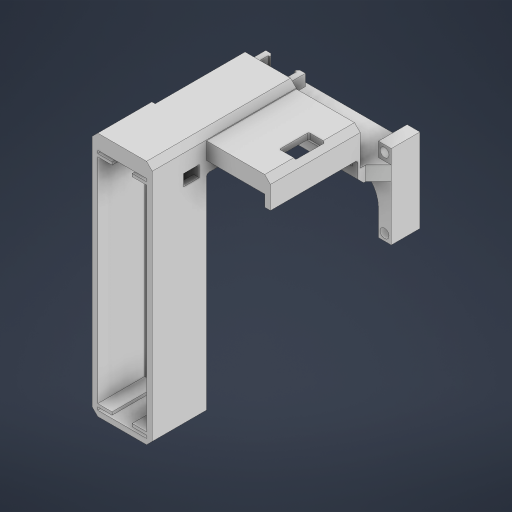
# Autodesk Inventor part: ElectronicsMount
Saved by Autodesk Inventor 2024.1 (Build 281209000, 209)
## iProperties
Created: 2023-11-16
Part Number: ElectronicsMount
Material: Generic
Document SubType Name: Modeling
Designer: Brandon
Density: 1 g/cm^3
Appearance: Default
Author: Brandon
Autodesk Inventor part; units mm, degrees
ref_plane "YZ Plane" through (0, 0, 0) normal (1, 0, 0) x (0, 1, 0)
ref_plane "XZ Plane" through (0, 0, 0) normal (0, 1, 0) x (-1, 0, 0)
sketch "Sketch1" plane through (0, 0, 0) normal (0, 0, 1) x (1, 0, 0)
  line L0 (-22, -8.75) -> (-22, 8.75) projected
  arc A0 (-22, -8.75) -> (-21.5, -9.25) centre (-21.5, -8.75) ccw projected
  line L1 (21.5, -9.25) -> (-21.5, -9.25) projected
  arc A1 (21.5, -9.25) -> (22, -8.75) centre (21.5, -8.75) ccw projected
  line L2 (22, 8.75) -> (22, -8.75) projected
  arc A2 (22, 8.75) -> (21.5, 9.25) centre (21.5, 8.75) ccw projected
  line L3 (-21.5, 9.25) -> (21.5, 9.25) projected
  arc A3 (-21.5, 9.25) -> (-22, 8.75) centre (-21.5, 8.75) ccw projected
  line L4 (-16.6675, -6.9225) -> (-17.1175, -6.4725) projected
  line L5 (-16.2175, -6.4725) -> (-16.6675, -6.9225) projected
  line L6 (-14.5625, -6.4725) -> (-16.2175, -6.4725) projected
  line L7 (-14.1125, -6.9225) -> (-14.5625, -6.4725) projected
  line L8 (-13.6625, -6.4725) -> (-14.1125, -6.9225) projected
  line L9 (-12.0075, -6.4725) -> (-13.6625, -6.4725) projected
  line L10 (-11.5575, -6.9225) -> (-12.0075, -6.4725) projected
  line L11 (-11.1075, -6.4725) -> (-11.5575, -6.9225) projected
  line L12 (-9.4525, -6.4725) -> (-11.1075, -6.4725) projected
  line L13 (-9.0025, -6.9225) -> (-9.4525, -6.4725) projected
  line L14 (-8.5525, -6.4725) -> (-9.0025, -6.9225) projected
  line L15 (-6.8975, -6.4725) -> (-8.5525, -6.4725) projected
  line L16 (-6.4475, -6.9225) -> (-6.8975, -6.4725) projected
  line L17 (-5.9975, -6.4725) -> (-6.4475, -6.9225) projected
  line L18 (-4.3425, -6.4725) -> (-5.9975, -6.4725) projected
  line L19 (-3.8925, -6.9225) -> (-4.3425, -6.4725) projected
  line L20 (-3.4425, -6.4725) -> (-3.8925, -6.9225) projected
  line L21 (-1.7875, -6.4725) -> (-3.4425, -6.4725) projected
  line L22 (-1.3375, -6.9225) -> (-1.7875, -6.4725) projected
  line L23 (-0.8875, -6.4725) -> (-1.3375, -6.9225) projected
  line L24 (0.7675, -6.4725) -> (-0.8875, -6.4725) projected
  line L25 (1.2175, -6.9225) -> (0.7675, -6.4725) projected
  line L26 (1.6675, -6.4725) -> (1.2175, -6.9225) projected
  line L27 (3.3225, -6.4725) -> (1.6675, -6.4725) projected
  line L28 (3.7725, -6.9225) -> (3.3225, -6.4725) projected
  line L29 (4.2225, -6.4725) -> (3.7725, -6.9225) projected
  line L30 (5.8775, -6.4725) -> (4.2225, -6.4725) projected
  line L31 (6.3275, -6.9225) -> (5.8775, -6.4725) projected
  line L32 (6.7775, -6.4725) -> (6.3275, -6.9225) projected
  line L33 (8.4325, -6.4725) -> (6.7775, -6.4725) projected
  line L34 (8.8825, -6.9225) -> (8.4325, -6.4725) projected
  line L35 (9.3325, -6.4725) -> (8.8825, -6.9225) projected
  line L36 (10.9875, -6.4725) -> (9.3325, -6.4725) projected
  line L37 (11.4375, -6.9225) -> (10.9875, -6.4725) projected
  line L38 (11.8875, -6.4725) -> (11.4375, -6.9225) projected
  line L39 (13.5425, -6.4725) -> (11.8875, -6.4725) projected
  line L40 (13.9925, -6.9225) -> (13.5425, -6.4725) projected
  line L41 (14.4425, -6.4725) -> (13.9925, -6.9225) projected
  line L42 (16.0975, -6.4725) -> (14.4425, -6.4725) projected
  line L43 (16.5475, -6.9225) -> (16.0975, -6.4725) projected
  line L44 (16.9975, -6.4725) -> (16.5475, -6.9225) projected
  line L45 (18.6525, -6.4725) -> (16.9975, -6.4725) projected
  line L46 (19.1025, -6.9225) -> (18.6525, -6.4725) projected
  line L47 (19.1025, -8.5775) -> (19.1025, -6.9225) projected
  line L48 (18.6525, -9.0275) -> (19.1025, -8.5775) projected
  line L49 (16.9975, -9.0275) -> (18.6525, -9.0275) projected
  line L50 (16.5475, -8.5775) -> (16.9975, -9.0275) projected
  line L51 (16.0975, -9.0275) -> (16.5475, -8.5775) projected
  line L52 (14.4425, -9.0275) -> (16.0975, -9.0275) projected
  line L53 (13.9925, -8.5775) -> (14.4425, -9.0275) projected
  line L54 (13.5425, -9.0275) -> (13.9925, -8.5775) projected
  line L55 (11.8875, -9.0275) -> (13.5425, -9.0275) projected
  line L56 (11.4375, -8.5775) -> (11.8875, -9.0275) projected
  line L57 (10.9875, -9.0275) -> (11.4375, -8.5775) projected
  line L58 (9.3325, -9.0275) -> (10.9875, -9.0275) projected
  line L59 (8.8825, -8.5775) -> (9.3325, -9.0275) projected
  line L60 (8.4325, -9.0275) -> (8.8825, -8.5775) projected
  line L61 (6.7775, -9.0275) -> (8.4325, -9.0275) projected
  line L62 (6.3275, -8.5775) -> (6.7775, -9.0275) projected
  line L63 (5.8775, -9.0275) -> (6.3275, -8.5775) projected
  line L64 (4.2225, -9.0275) -> (5.8775, -9.0275) projected
  line L65 (3.7725, -8.5775) -> (4.2225, -9.0275) projected
  line L66 (3.3225, -9.0275) -> (3.7725, -8.5775) projected
  line L67 (1.6675, -9.0275) -> (3.3225, -9.0275) projected
  line L68 (1.2175, -8.5775) -> (1.6675, -9.0275) projected
  line L69 (0.7675, -9.0275) -> (1.2175, -8.5775) projected
  line L70 (-0.8875, -9.0275) -> (0.7675, -9.0275) projected
  line L71 (-1.3375, -8.5775) -> (-0.8875, -9.0275) projected
  line L72 (-1.7875, -9.0275) -> (-1.3375, -8.5775) projected
  line L73 (-3.4425, -9.0275) -> (-1.7875, -9.0275) projected
  line L74 (-3.8925, -8.5775) -> (-3.4425, -9.0275) projected
  line L75 (-4.3425, -9.0275) -> (-3.8925, -8.5775) projected
  line L76 (-5.9975, -9.0275) -> (-4.3425, -9.0275) projected
  line L77 (-6.4475, -8.5775) -> (-5.9975, -9.0275) projected
  line L78 (-6.8975, -9.0275) -> (-6.4475, -8.5775) projected
  line L79 (-8.5525, -9.0275) -> (-6.8975, -9.0275) projected
  line L80 (-9.0025, -8.5775) -> (-8.5525, -9.0275) projected
  line L81 (-9.4525, -9.0275) -> (-9.0025, -8.5775) projected
  line L82 (-11.1075, -9.0275) -> (-9.4525, -9.0275) projected
  line L83 (-11.5575, -8.5775) -> (-11.1075, -9.0275) projected
  line L84 (-12.0075, -9.0275) -> (-11.5575, -8.5775) projected
  line L85 (-13.6625, -9.0275) -> (-12.0075, -9.0275) projected
  line L86 (-14.1125, -8.5775) -> (-13.6625, -9.0275) projected
  line L87 (-14.5625, -9.0275) -> (-14.1125, -8.5775) projected
  line L88 (-16.2175, -9.0275) -> (-14.5625, -9.0275) projected
  line L89 (-16.6675, -8.5775) -> (-16.2175, -9.0275) projected
  line L90 (-17.1175, -9.0275) -> (-16.6675, -8.5775) projected
  line L91 (-18.7725, -9.0275) -> (-17.1175, -9.0275) projected
  line L92 (-19.2225, -8.5775) -> (-18.7725, -9.0275) projected
  line L93 (-19.2225, -6.9225) -> (-19.2225, -8.5775) projected
  line L94 (-18.7725, -6.4725) -> (-19.2225, -6.9225) projected
  line L95 (-17.1175, -6.4725) -> (-18.7725, -6.4725) projected
  circle A4 centre (-20.5, 7.75) radius 1 projected
  circle A5 centre (20.5, 7.75) radius 1 projected
  circle A6 centre (20.5, -7.75) radius 1 projected
  circle A7 centre (-20.5, -7.75) radius 1 projected
  circle A8 centre (18.5, 2) radius 0.5 projected
  circle A9 centre (18.5, 0) radius 0.5 projected
  circle A10 centre (18.5, -2) radius 0.5 projected
  circle A11 centre (20.25, 2) radius 0.5 projected
  circle A12 centre (20.25, 0) radius 0.5 projected
  circle A13 centre (20.25, -2) radius 0.5 projected
  line L96 (16.9975, 6.4725) -> (16.5475, 6.9225) projected
  line L97 (16.5475, 6.9225) -> (16.0975, 6.4725) projected
  line L98 (16.0975, 6.4725) -> (14.4425, 6.4725) projected
  line L99 (14.4425, 6.4725) -> (13.9925, 6.9225) projected
  line L100 (13.9925, 6.9225) -> (13.5425, 6.4725) projected
  line L101 (13.5425, 6.4725) -> (11.8875, 6.4725) projected
  line L102 (11.8875, 6.4725) -> (11.4375, 6.9225) projected
  line L103 (11.4375, 6.9225) -> (10.9875, 6.4725) projected
  line L104 (10.9875, 6.4725) -> (9.3325, 6.4725) projected
  line L105 (9.3325, 6.4725) -> (8.8825, 6.9225) projected
  line L106 (8.8825, 6.9225) -> (8.4325, 6.4725) projected
  line L107 (8.4325, 6.4725) -> (6.7775, 6.4725) projected
  line L108 (6.7775, 6.4725) -> (6.3275, 6.9225) projected
  line L109 (6.3275, 6.9225) -> (5.8775, 6.4725) projected
  line L110 (5.8775, 6.4725) -> (4.2225, 6.4725) projected
  line L111 (4.2225, 6.4725) -> (3.7725, 6.9225) projected
  line L112 (3.7725, 6.9225) -> (3.3225, 6.4725) projected
  line L113 (3.3225, 6.4725) -> (1.6675, 6.4725) projected
  line L114 (1.6675, 6.4725) -> (1.2175, 6.9225) projected
  line L115 (1.2175, 6.9225) -> (0.7675, 6.4725) projected
  line L116 (0.7675, 6.4725) -> (-0.8875, 6.4725) projected
  line L117 (-0.8875, 6.4725) -> (-1.3375, 6.9225) projected
  line L118 (-1.3375, 6.9225) -> (-1.7875, 6.4725) projected
  line L119 (-1.7875, 6.4725) -> (-3.4425, 6.4725) projected
  line L120 (-3.4425, 6.4725) -> (-3.8925, 6.9225) projected
  line L121 (-3.8925, 6.9225) -> (-4.3425, 6.4725) projected
  line L122 (-4.3425, 6.4725) -> (-5.9975, 6.4725) projected
  line L123 (-5.9975, 6.4725) -> (-6.4475, 6.9225) projected
  line L124 (-6.4475, 6.9225) -> (-6.8975, 6.4725) projected
  line L125 (-6.8975, 6.4725) -> (-8.5525, 6.4725) projected
  line L126 (-8.5525, 6.4725) -> (-9.0025, 6.9225) projected
  line L127 (-9.0025, 6.9225) -> (-9.4525, 6.4725) projected
  line L128 (-9.4525, 6.4725) -> (-11.1075, 6.4725) projected
  line L129 (-11.1075, 6.4725) -> (-11.5575, 6.9225) projected
  line L130 (-11.5575, 6.9225) -> (-12.0075, 6.4725) projected
  line L131 (-12.0075, 6.4725) -> (-13.6625, 6.4725) projected
  line L132 (-13.6625, 6.4725) -> (-14.1125, 6.9225) projected
  line L133 (-14.1125, 6.9225) -> (-14.5625, 6.4725) projected
  line L134 (-14.5625, 6.4725) -> (-16.2175, 6.4725) projected
  line L135 (-16.2175, 6.4725) -> (-16.6675, 6.9225) projected
  line L136 (-16.6675, 6.9225) -> (-17.1175, 6.4725) projected
  line L137 (-17.1175, 6.4725) -> (-18.7725, 6.4725) projected
  line L138 (-18.7725, 6.4725) -> (-19.2225, 6.9225) projected
  line L139 (-19.2225, 6.9225) -> (-19.2225, 8.5775) projected
  line L140 (-19.2225, 8.5775) -> (-18.7725, 9.0275) projected
  line L141 (-18.7725, 9.0275) -> (-17.1175, 9.0275) projected
  line L142 (-17.1175, 9.0275) -> (-16.6675, 8.5775) projected
  line L143 (-16.6675, 8.5775) -> (-16.2175, 9.0275) projected
  line L144 (-16.2175, 9.0275) -> (-14.5625, 9.0275) projected
  line L145 (-14.5625, 9.0275) -> (-14.1125, 8.5775) projected
  line L146 (-14.1125, 8.5775) -> (-13.6625, 9.0275) projected
  line L147 (-13.6625, 9.0275) -> (-12.0075, 9.0275) projected
  line L148 (-12.0075, 9.0275) -> (-11.5575, 8.5775) projected
  line L149 (-11.5575, 8.5775) -> (-11.1075, 9.0275) projected
  line L150 (-11.1075, 9.0275) -> (-9.4525, 9.0275) projected
  line L151 (-9.4525, 9.0275) -> (-9.0025, 8.5775) projected
  line L152 (-9.0025, 8.5775) -> (-8.5525, 9.0275) projected
  line L153 (-8.5525, 9.0275) -> (-6.8975, 9.0275) projected
  line L154 (-6.8975, 9.0275) -> (-6.4475, 8.5775) projected
  line L155 (-6.4475, 8.5775) -> (-5.9975, 9.0275) projected
  line L156 (-5.9975, 9.0275) -> (-4.3425, 9.0275) projected
  line L157 (-4.3425, 9.0275) -> (-3.8925, 8.5775) projected
  line L158 (-3.8925, 8.5775) -> (-3.4425, 9.0275) projected
  line L159 (-3.4425, 9.0275) -> (-1.7875, 9.0275) projected
  line L160 (-1.7875, 9.0275) -> (-1.3375, 8.5775) projected
  line L161 (-1.3375, 8.5775) -> (-0.8875, 9.0275) projected
  line L162 (-0.8875, 9.0275) -> (0.7675, 9.0275) projected
  line L163 (0.7675, 9.0275) -> (1.2175, 8.5775) projected
  line L164 (1.2175, 8.5775) -> (1.6675, 9.0275) projected
  line L165 (1.6675, 9.0275) -> (3.3225, 9.0275) projected
  line L166 (3.3225, 9.0275) -> (3.7725, 8.5775) projected
  line L167 (3.7725, 8.5775) -> (4.2225, 9.0275) projected
  line L168 (4.2225, 9.0275) -> (5.8775, 9.0275) projected
  line L169 (5.8775, 9.0275) -> (6.3275, 8.5775) projected
  line L170 (6.3275, 8.5775) -> (6.7775, 9.0275) projected
  line L171 (6.7775, 9.0275) -> (8.4325, 9.0275) projected
  line L172 (8.4325, 9.0275) -> (8.8825, 8.5775) projected
  line L173 (8.8825, 8.5775) -> (9.3325, 9.0275) projected
  line L174 (9.3325, 9.0275) -> (10.9875, 9.0275) projected
  line L175 (10.9875, 9.0275) -> (11.4375, 8.5775) projected
  line L176 (11.4375, 8.5775) -> (11.8875, 9.0275) projected
  line L177 (11.8875, 9.0275) -> (13.5425, 9.0275) projected
  line L178 (13.5425, 9.0275) -> (13.9925, 8.5775) projected
  line L179 (13.9925, 8.5775) -> (14.4425, 9.0275) projected
  line L180 (14.4425, 9.0275) -> (16.0975, 9.0275) projected
  line L181 (16.0975, 9.0275) -> (16.5475, 8.5775) projected
  line L182 (16.5475, 8.5775) -> (16.9975, 9.0275) projected
  line L183 (16.9975, 9.0275) -> (18.6525, 9.0275) projected
  line L184 (18.6525, 9.0275) -> (19.1025, 8.5775) projected
  line L185 (19.1025, 8.5775) -> (19.1025, 6.9225) projected
  line L186 (19.1025, 6.9225) -> (18.6525, 6.4725) projected
  line L187 (18.6525, 6.4725) -> (16.9975, 6.4725) projected
  line L188 (19.1533, 9.25) -> (22, 9.25)
  line L189 (22, 9.25) -> (22, -9.25)
  line L190 (22, -9.25) -> (19.1533, -9.25)
  line L191 (19.1533, -9.25) -> (19.1533, 9.25)
  line L192 (19.1533, 6.0915) -> (-6.3742, 6.0915)
  line L193 (-6.3742, 6.0915) -> (-6.3742, 2.9063)
  line L194 (-6.3742, 2.9063) -> (19.1533, 2.9063)
  line L195 (19.1533, 2.9063) -> (19.1533, 6.0915)
  line L196 (-6.3742, 7.9898) -> (-6.3742, 13.378) projected
  point P0 (0, 0)
  point P1 (19.1533, 2.9063)
  point P2 (21.5, 9.25)
  dimension "d0" = 0.0508
  dimension "d1" = 3.1852
  dimension "d2" = 0.381
  constraints: 16 end point, 4 parallel, 3 point on line, 2 horizontal, 2 perpendicular, 2 vertical alignment
  measures "d0" distance between parallel lines of L185 L191
  measures "d1" distance of L193.end L192.end
  measures "d2" distance between parallel lines of L187 L192
extrude "Extrusion1" add sketch "Sketch1" along normal blind 6.35 contours L191 L3 A2 L2 A1 L1 | A1 L189 L190 | L194 L193 L192 L191 | L188 L189 A2 | A11 | A12 | A13
extrude "Extrusion2" add sketch "Sketch1" along normal blind 10.8966 contours L194 L193 L192 L191
ref_plane "Work Plane1" through (5.2995, -4.5055, 30.861) normal (-1, 0, 0) x (0, 0, 1)
sketch "Sketch2" plane through (5.2995, -4.5055, 30.861) normal (-1, 0, 0) x (0, 0, 1)
  line L0 (-20.4794, 19.9727) -> (-20.4794, 14.2727) projected
  line L1 (-23.7794, 14.1227) -> (-20.4794, 14.1227) projected
  line L2 (-20.4794, 14.1227) -> (-20.4794, 14.2727) projected
  line L3 (-22.861, 12.2055) -> (-22.861, 12.3055) projected
  line L4 (-24.511, 10.597) -> (-24.511, 7.4119) projected
  line L5 (-24.511, 10.597) -> (-19.9644, 10.597) projected
  line L6 (-19.9644, 7.4119) -> (-19.9644, 10.597) projected
  line L7 (-24.511, 7.4119) -> (-19.9644, 7.4119) projected
  line L8 (-1.2709, 12.3491) -> (-19.3031, 12.3491) projected
  line L9 (-19.9644, 10.597) -> (-19.9644, 12.3999)
  line L10 (-19.9644, 12.3999) -> (-0.5877, 12.3999)
  line L11 (-19.9644, 12.3999) -> (-0.5877, 12.3999) construction
  line L12 (-22.734, 14.1227) -> (-22.734, 10.597)
  line L13 (-20.4794, 19.9727) -> (-20.4794, 20.1227) projected
  line L14 (-20.4794, 20.1227) -> (11.4051, 20.1227)
  line L15 (7.2801, 15.1429) -> (5.2801, 15.1429) projected
  line L16 (-0.5877, 12.3999) -> (-0.5877, -34.2331)
  line L17 (4.0301, -29.2071) -> (8.5301, -29.2071) projected
  line L18 (-3.8264, -34.2331) -> (-1.587, -34.2331) projected
  line L19 (-0.6385, 11.6992) -> (-0.6385, -27.2331) projected
  line L20 (0.9998, 16.8447) -> (0.9998, -33.0171)
  line L21 (0.9998, 16.8447) -> (11.4051, 16.8447)
  line L22 (11.4051, 13.1429) -> (11.4051, 0.3429)
  line L23 (11.4051, 16.8447) -> (11.4051, 20.1227)
  line L24 (0.9998, -33.0171) -> (11.4051, -33.0171)
  line L25 (-0.5877, -34.2331) -> (11.4051, -34.2331)
  line L26 (11.4051, -34.2331) -> (11.4051, -33.0171)
  line L27 (11.4051, -33.0171) -> (11.4051, 16.8447)
  line L28 (-0.5877, 12.3999) -> (-0.5877, 20.1227)
  point P0 (-30.861, 4.5055)
  point P1 (-0.5877, 12.3999)
  point P2 (11.4051, 0.3429)
  dimension "d7" = 0.0508
  dimension "d8" = 0
  dimension "d9" = 0.127
  dimension "d10" = 0.0508
  dimension "d11" = 1.5875
  dimension "d12" = 1.7018
  dimension "d13" = 3.81
  constraints: 31 end point, 5 horizontal, 5 vertical, 4 point on line, 3 perpendicular, 2 vertical alignment, 1 collinear, 1 horizontal alignment, 1 parallel, 2 other
  measures "d7" vertical distance of L9.end L8.end
  measures "d8" distance between parallel lines of L10 L11
  measures "d9" distance between parallel lines of L12 L3
  measures "d10" distance between parallel lines of L19 L16
  measures "d11" distance between parallel lines of L16 L20
  measures "d12" distance from line of L20.start L15
  measures "d13" distance between parallel lines of L24 L17
extrude "Extrusion3" add sketch "Sketch2" along normal blind 1.5875 contours L13 L14 L28 L10 L9 L5 L12 L1 L2 L0 | L14 L23 L21 L20 L24 L26 L25 L16 L28 | L27 L22 L24 L20 L21
extrude "Extrusion4" add sketch "Sketch2" along normal blind 11.6586 contours L13 L14 L28 L10 L9 L5 L12 L1 L2 L0 | L14 L23 L21 L20 L24 L26 L25 L16 L28
extrude "Extrusion5" add sketch "Sketch2" along normal blind 12.3952 contours L14 L23 L21 L20 L24 L26 L25 L16 L28
sketch "Sketch3" plane through (-7.0957, -4.5055, 30.861) normal (-1, 0, 0) x (0, 0, 1)
  line L0 (-19.9644, 12.3999) -> (-0.5877, 12.3999) projected
  line L1 (-19.9644, 10.597) -> (-19.9644, 12.3999) projected
  line L2 (-22.734, 10.597) -> (-19.9644, 10.597) projected
  line L3 (-22.734, 14.1227) -> (-22.734, 10.597) projected
  line L4 (-20.4794, 14.1227) -> (-22.734, 14.1227) projected
  line L5 (-20.4794, 20.1227) -> (-20.4794, 14.1227) projected
  line L6 (11.4051, 20.1227) -> (-20.4794, 20.1227) projected
  line L7 (11.4051, -34.2331) -> (11.4051, 20.1227) projected
  line L8 (-0.5877, -34.2331) -> (11.4051, -34.2331) projected
  line L9 (-0.5877, 12.3999) -> (-0.5877, -34.2331) projected
  line L10 (-0.5877, 12.3999) -> (-0.5877, 20.1227) projected
  point P0 (-30.861, 4.5055)
  point P1 (-17.4793, -0.0169)
  constraints: 1 other
extrude "Extrusion6" add sketch "Sketch3" along normal blind 1.27 contours L10 L6 L7 L8 L9
extrude "Extrusion7" cut sketch "Sketch2" along normal blind 0.3175 contours L13 L14 L28 L10 L9 L5 L12 L1 L2 L0 | L14 L23 L21 L20 L24 L26 L25 L16 L28 | L27 L22 L24 L20 L21
sketch "Sketch4" plane through (-8.3657, -38.7386, 42.2661) normal (0, 0, 1) x (1, 0, 0)
  line L0 (13.3477, 0) -> (13.3477, 54.3558) projected
  line L1 (13.3477, 54.3558) -> (0, 54.3558) projected
  line L2 (0, 0) -> (0, 54.3558) projected
  line L3 (13.3477, 0) -> (0, 0) projected
  line L4 (12.0777, 51.0778) -> (1.27, 51.0778) projected
  line L5 (12.0777, 1.216) -> (12.0777, 51.0778) projected
  line L6 (12.0777, 1.216) -> (1.27, 1.216) projected
  line L7 (1.27, 1.216) -> (1.27, 51.0778) projected
  line L8 (1.27, 1.216) -> (12.0777, 1.216)
  line L9 (12.0777, 1.216) -> (12.0777, 1.851)
  line L10 (12.0777, 1.851) -> (1.27, 1.851)
  line L11 (1.27, 1.851) -> (1.27, 1.216)
  line L12 (1.27, 1.851) -> (12.0777, 1.851)
  line L13 (12.0777, 1.851) -> (12.0777, 2.486)
  line L14 (12.0777, 2.486) -> (1.27, 2.486)
  line L15 (1.27, 2.486) -> (1.27, 1.851)
  line L16 (4.4514, 2.486) -> (8.8964, 2.486)
  line L17 (8.8964, 2.486) -> (8.8964, 1.851)
  line L18 (8.8964, 1.851) -> (4.4514, 1.851)
  line L19 (4.4514, 1.851) -> (4.4514, 2.486)
  line L20 (1.27, 51.0778) -> (12.0777, 51.0778)
  line L21 (12.0777, 51.0778) -> (12.0777, 50.4428)
  line L22 (12.0777, 50.4428) -> (1.27, 50.4428)
  line L23 (1.27, 50.4428) -> (1.27, 51.0778)
  line L24 (1.27, 50.4428) -> (12.0777, 50.4428)
  line L25 (12.0777, 50.4428) -> (12.0777, 49.8078)
  line L26 (12.0777, 49.8078) -> (1.27, 49.8078)
  line L27 (1.27, 49.8078) -> (1.27, 50.4428)
  line L28 (4.4514, 50.4428) -> (8.8964, 50.4428)
  line L29 (8.8964, 50.4428) -> (8.8964, 49.8078)
  line L30 (8.8964, 49.8078) -> (4.4514, 49.8078)
  line L31 (4.4514, 49.8078) -> (4.4514, 50.4428)
  point P0 (8.3657, 38.7386)
  point P1 (6.6739, 2.486)
  point P2 (6.6739, 50.4428)
  point P3 (6.6739, 50.4428)
  point P4 (8.8964, 1.851)
  point P5 (4.4514, 1.851)
  point P6 (1.27, 2.486)
  point P7 (1.27, 1.851)
  point P8 (1.27, 50.4428)
  point P9 (1.27, 49.8078)
  dimension "d24" = 0.635
  dimension "d25" = 0.635
  dimension "d26" = 4.445
  dimension "d27" = 0.635
  dimension "d28" = 0.635
  dimension "d29" = 4.445
  constraints: 48 end point, 12 parallel, 8 point on line, 6 horizontal, 6 perpendicular, 4 midpoint, 1 coincident
  measures "d24" distance of L9.end L8.end
  measures "d25" distance of L13.end L12.end
  measures "d26" distance of L17.end L18.end
  measures "d27" distance of L20.end L21.end
  measures "d28" distance of L24.end L25.end
  measures "d29" distance of L29.end L30.end
extrude "Extrusion8" add sketch "Sketch4" against normal up to surface (10.4053 mm away) contours L5 L26 L29 L22 | L22 L31 L26 L7 | L5 L10 L17 L14 | L14 L19 L10 L7
sketch "Sketch5" plane through (4.982, -4.5055, 30.861) normal (1, 0, 0) x (0, 0, -1)
  line L0 (20.4794, 20.1227) -> (20.4794, 14.1227) projected
  line L1 (-11.4051, 20.1227) -> (20.4794, 20.1227) projected
  line L2 (-11.4051, -34.2331) -> (-11.4051, 20.1227) projected
  line L3 (0.5877, -34.2331) -> (-11.4051, -34.2331) projected
  line L4 (0.5877, 12.3999) -> (0.5877, -34.2331) projected
  line L5 (19.9644, 12.3999) -> (0.5877, 12.3999) projected
  line L6 (19.9644, 10.597) -> (19.9644, 12.3999) projected
  line L7 (22.734, 10.597) -> (19.9644, 10.597) projected
  line L8 (22.734, 14.1227) -> (22.734, 10.597) projected
  line L9 (20.4794, 14.1227) -> (22.734, 14.1227) projected
  line L10 (0.5877, 20.1227) -> (0.5877, 14.9399)
  line L11 (0.5877, 12.3999) -> (0.5877, 20.1227) projected
  line L12 (0.5877, 14.9399) -> (1.8577, 14.9399)
  line L13 (1.8577, 14.9399) -> (1.8577, 17.4135)
  line L14 (1.8577, 17.4135) -> (20.4794, 17.4135)
  line L15 (19.2094, 17.4135) -> (19.2094, 14.9399)
  line L16 (19.2094, 14.9399) -> (20.4794, 14.9399)
  line L17 (6.6976, 18.6835) -> (13.8764, 18.6835) projected
  line L18 (0.5877, 18.6835) -> (6.6976, 18.6835)
  line L19 (13.8764, 18.6835) -> (20.4794, 18.6835)
  line L20 (0.5877, 14.9399) -> (-4.4923, 14.9399)
  line L21 (-4.4923, 14.9399) -> (-4.4923, 12.3999)
  line L22 (-4.4923, 12.3999) -> (0.5877, 12.3999)
  line L23 (0.5877, 12.3999) -> (0.5877, 14.9399)
  line L24 (-0.9998, -33.0171) -> (-0.9998, -32.3821) projected
  line L25 (-0.9998, -32.3821) -> (-0.9998, -33.0171) projected
  line L26 (-0.9998, -32.3821) -> (-0.9998, -31.7471) projected
  line L27 (-0.9998, 15.5747) -> (-0.9998, -31.7471) projected
  line L28 (-0.9998, 15.5747) -> (-0.9998, 16.2097) projected
  line L29 (-0.9998, 16.8447) -> (-0.9998, 16.2097) projected
  line L30 (-0.9998, 16.2097) -> (-0.9998, 16.8447) projected
  line L31 (-0.9998, 16.2097) -> (-0.9998, 15.5747) projected
  line L32 (-0.9998, -31.7471) -> (-0.9998, 15.5747) projected
  line L33 (-0.9998, -31.7471) -> (-0.9998, -32.3821) projected
  point P0 (30.861, 4.5055)
  point P1 (-0.9998, 12.3999)
  point P2 (-0.9998, 14.9399)
  dimension "d32" = 2.54
  dimension "d33" = 1.27
  dimension "d35" = 1.27
  dimension "d36" = 1.27
  dimension "d43" = 5.08
  constraints: 24 end point, 8 point on line, 6 perpendicular, 2 horizontal, 2 horizontal alignment, 2 parallel
  measures "d32" distance from line of L10.end L5
  measures "d33" distance of L10.end L12.end
  measures "d35" distance between parallel lines of L0 L15
  measures "d36" distance between parallel lines of L17 L14
  measures "d43" distance of L22.end L21.end
extrude "Extrusion9" add sketch "Sketch5" along normal up to surface (14.1713 mm away) contours L0 L14 L13 L12 L10 L18 L17 L19 | L0 L16 L15 L14
sketch "Sketch6" plane through (19.1533, 2.9063, 6.35) normal (1, 0, 0) x (0, 0, -1)
  line L0 (-4.0316, 7.528) -> (-5.3016, 7.528) projected
  line L1 (-5.3016, 7.528) -> (-5.3016, 10.0016) projected
  line L2 (-5.3016, 10.0016) -> (-22.6533, 10.0016) projected
  line L3 (-22.6533, 10.0016) -> (-22.6533, 7.528) projected
  line L4 (-22.6533, 7.528) -> (-23.9233, 7.528) projected
  line L5 (-23.9233, 7.528) -> (-23.9233, 11.2716) projected
  line L6 (-23.9233, 11.2716) -> (-4.0316, 11.2716) projected
  line L7 (-4.0316, 12.7108) -> (-4.0316, 11.2716) projected
  line L8 (-35.9161, 12.7108) -> (-4.0316, 12.7108) projected
  line L9 (-35.9161, -41.645) -> (-35.9161, 12.7108) projected
  line L10 (-23.9233, -41.645) -> (-35.9161, -41.645) projected
  line L11 (-23.9233, 4.988) -> (-23.9233, -41.645) projected
  line L12 (-4.5466, 4.988) -> (-23.9233, 4.988) projected
  line L13 (-4.5466, 3.1852) -> (-4.5466, 4.988) projected
  line L14 (-1.777, 3.1852) -> (-4.5466, 3.1852) projected
  line L15 (-1.777, 6.7108) -> (-1.777, 3.1852) projected
  line L16 (-4.0316, 6.7108) -> (-1.777, 6.7108) projected
  line L17 (-4.0316, 7.528) -> (-4.0316, 6.7108) projected
  line L18 (-4.0316, 11.2716) -> (-4.0316, 7.528) projected
  line L19 (-23.9233, 7.528) -> (-23.9233, 4.988)
  point P0 (6.35, -2.9063)
  constraints: 2 end point, 1 vertical
extrude "Extrusion10" add sketch "Sketch6" against normal blind 1.27 contours L17 L16 L15 L14 L13 L12 L19 L4 L3 L2 L1 L0 | L0 L1 L2 L3 L4 L5 L6 L18
sketch "Sketch7" plane through (4.982, 14.178, 30.2733) normal (0, 1, 0) x (1, 0, 0)
  line L0 (-8.8562, 0.6832) -> (-8.8562, 18.7155) projected
  line L1 (11.1938, 0.6832) -> (-8.8562, 0.6832) projected
  line L2 (11.1938, 0.6832) -> (11.1938, 5.6065) projected
  line L3 (11.1938, 5.9493) -> (11.1938, 5.6065) projected
  line L4 (9.6938, 5.9493) -> (11.1938, 5.9493) projected
  ellipse E0 centre (9.6938, 6.4493) end of major axis (9.6938, 5.9493) minor radius 0.5 (9.1938, 6.4493) -> (9.6938, 5.9493) ccw projected
  line L5 (9.1938, 12.9493) -> (9.1938, 6.4493) projected
  ellipse E1 centre (9.6938, 12.9493) end of major axis (9.6938, 12.4493) minor radius 0.5 (9.6938, 13.4493) -> (9.1938, 12.9493) ccw projected
  line L6 (11.1938, 13.4493) -> (9.6938, 13.4493) projected
  line L7 (11.1938, 13.7933) -> (11.1938, 13.4493) projected
  line L8 (11.1938, 18.7155) -> (11.1938, 13.7933) projected
  line L9 (11.1938, 18.7155) -> (-8.8562, 18.7155) projected
  line L10 (11.1938, 5.9493) -> (11.1938, 5.6065) projected
  line L11 (11.3438, 5.6065) -> (11.1938, 5.6065) projected
  line L12 (11.3438, 0.6832) -> (11.3438, 5.6065) projected
  line L13 (13.1938, 0.6832) -> (11.3438, 0.6832) projected
  line L14 (13.1938, 6.7493) -> (13.1938, 0.6832) projected
  arc A0 (12.8938, 6.4493) -> (13.1938, 6.7493) centre (12.8938, 6.7493) ccw projected
  line L15 (9.9938, 6.4493) -> (12.8938, 6.4493) projected
  arc A1 (9.6938, 6.7493) -> (9.9938, 6.4493) centre (9.9938, 6.7493) ccw projected
  line L16 (9.6938, 12.6493) -> (9.6938, 6.7493) projected
  arc A2 (9.9938, 12.9493) -> (9.6938, 12.6493) centre (9.9938, 12.6493) ccw projected
  line L17 (12.8938, 12.9493) -> (9.9938, 12.9493) projected
  arc A3 (13.1938, 12.6493) -> (12.8938, 12.9493) centre (12.8938, 12.6493) ccw projected
  line L18 (13.1938, 18.7155) -> (13.1938, 12.6493) projected
  line L19 (13.1938, 18.7155) -> (11.3438, 18.7155) projected
  line L20 (11.3438, 13.7933) -> (11.3438, 18.7155) projected
  line L21 (11.3438, 13.7933) -> (11.1938, 13.7933) projected
  line L22 (11.1938, 13.7933) -> (11.1938, 13.4493) projected
  line L23 (11.1938, 13.4493) -> (9.6938, 13.4493) projected
  arc A4 (9.6938, 13.4493) -> (9.1938, 12.9493) centre (9.6938, 12.9493) ccw projected
  line L24 (9.1938, 12.9493) -> (9.1938, 6.4493) projected
  arc A5 (9.1938, 6.4493) -> (9.6938, 5.9493) centre (9.6938, 6.4493) ccw projected
  line L25 (9.6938, 5.9493) -> (11.1938, 5.9493) projected
  line L26 (13.1938, 6.7493) -> (13.1938, 12.6493)
  point P0 (-4.982, 30.2733)
  constraints: 2 end point, 1 vertical, 2 other
extrude "Extrusion11" cut sketch "Sketch7" against normal through all contours A0 L15 A1 L16 A2 L17 A3 L26
extrude "Extrusion12" cut sketch "Sketch5" against normal blind 2.54 contours L27 L22 L21 L20
chamfer "Chamfer1" distance 1.27 angle 45 8 edges at (4.982, -38.7386, 36.2697) (-8.3657, -38.7386, 36.2697) (-8.3657, 15.6171, 36.2697) (4.982, 15.6171, 26.3239) (18.5183, 9.6171, 8.127) (6.3895, 2.9063, 10.8966) (19.1533, 14.178, 20.3275) (-6.3742, 2.9063, 5.4483)
fillet "Fillet2" radius 6.35 1 edges at (19.1533, 2.9063, 3.175)
chamfer "Chamfer2" distance 2.8448 angle 45 1 edges at (19.1533, 4.4989, 6.35)
sketch "Sketch8" plane through (17.8833, 9.6171, 10.3816) normal (0, 1, 0) x (1, 0, 0)
  line L0 (0, 0.9846) -> (1.27, 0.9846) projected
  line L1 (0, 0) -> (0, 0.9846) projected
  line L2 (1.27, 0) -> (0, 0) projected
  line L3 (1.27, 0.9846) -> (1.27, 0) projected
  line L4 (0, 2.2546) -> (0, 0.9846) projected
  line L5 (0, 0.9846) -> (1.27, 0.9846) projected
  line L6 (1.27, 0.9846) -> (1.27, 1.1868) projected
  line L7 (1.27, 1.1868) -> (2.3378, 2.2546) projected
  line L8 (2.3378, 2.2546) -> (0, 2.2546) projected
  point P0 (-17.8833, 10.3816)
  point P1 (0, 0.9846)
  point P2 (1.27, 0.9846)
extrude "Extrusion13" cut sketch "Sketch8" against normal blind 3.5256
fillet "Fillet3" radius 0.635 3 edges at (18.5183, 7.8943, 10.8966) (-0.6886, 7.8943, 10.8966) (-0.6886, 7.8943, 30.2733)
sketch "Sketch9" plane through (-6.3591, -4.5055, 30.861) normal (-1, 0, 0) x (0, 0, 1)
  arc A0 (-16.68, 18.5098) -> (-13.944, 18.5098) centre (-15.312, 17.0167) ccw projected
  arc A1 (-6.63, 18.5098) -> (-3.894, 18.5098) centre (-5.262, 17.0167) ccw projected
  circle A2 centre (-15.312, 17.0167) radius 2.025
  circle A3 centre (-5.262, 17.0167) radius 2.025
  point P0 (-30.861, 4.5055)
  point P1 (-6.63, 18.5098)
  constraints: 2 coincident, 6 other
extrude "Extrusion14" cut sketch "Sketch9" against normal blind 8.89
chamfer "Chamfer3" distance 0.254 angle 45 2 edges at (-6.3591, 11.0181, 14.181) (-6.3591, 11.0181, 24.231)
sketch "Sketch10" plane through (-6.3591, 9.6171, 10.3816) normal (0, 0, -1) x (-1, 0, 0)
  line L0 (-1.6673, 0.15) -> (-1.6673, 5.85) projected
  arc A0 (-1.6673, 5.85) -> (-1.8173, 6) centre (-1.8173, 5.85) ccw projected
  line L1 (-1.8173, 6) -> (-7.5173, 6) projected
  arc A1 (-7.5173, 6) -> (-7.6673, 5.85) centre (-7.5173, 5.85) ccw projected
  line L2 (-7.6673, 5.85) -> (-7.6673, 0.15) projected
  arc A2 (-7.6673, 0.15) -> (-7.5173, 0) centre (-7.5173, 0.15) ccw projected
  line L3 (-7.5173, 0) -> (-1.8173, 0) projected
  arc A3 (-1.8173, 0) -> (-1.6673, 0.15) centre (-1.8173, 0.15) ccw projected
  circle A4 centre (-2.4173, 0.75) radius 0.4 projected
  circle A5 centre (-6.9173, 5.25) radius 0.4 projected
  circle A6 centre (-6.9173, 0.75) radius 0.4 projected
  circle A7 centre (-2.4173, 5.25) radius 0.4 projected
  circle A8 centre (-4.6673, 3) radius 1.85 projected
  line L4 (-7.7943, 0.15) -> (-7.7943, 5.85)
  arc A9 (-7.5172, 6.127) -> (-7.7943, 5.85) centre (-7.5173, 5.85) ccw
  line L5 (-7.5172, 6.127) -> (-1.8173, 6.127)
  arc A10 (-1.5403, 5.85) -> (-1.8173, 6.127) centre (-1.8173, 5.85) ccw
  line L6 (-1.5403, 5.85) -> (-1.5403, 0.15)
  arc A11 (-1.8173, -0.127) -> (-1.5403, 0.15) centre (-1.8173, 0.15) ccw
  line L7 (-1.8173, -0.127) -> (-7.5172, -0.127)
  arc A12 (-7.7943, 0.15) -> (-7.5172, -0.127) centre (-7.5173, 0.15) ccw
  line L8 (-7.7943, 4.27) -> (-9.0643, 4.27)
  line L9 (-9.0643, 4.27) -> (-9.0643, 1.73)
  line L10 (-9.0643, 1.73) -> (-7.7943, 1.73)
  line L11 (-7.7943, 1.73) -> (-7.7943, 4.27)
  line L12 (-1.5403, 4.27) -> (-0.2703, 4.27)
  line L13 (-0.2703, 4.27) -> (-0.2703, 1.73)
  line L14 (-0.2703, 1.73) -> (-1.5403, 1.73)
  line L15 (-1.5403, 1.73) -> (-1.5403, 4.27)
  point P0 (-6.3591, -9.6171)
  point P1 (-7.7943, 3)
  point P2 (-1.5403, 3)
  point P3 (-1.5403, 1.73)
  point P4 (-7.7943, 1.73)
  dimension "d62" = 0.127
  dimension "d63" = 1.27
  dimension "d64" = 2.54
  dimension "d65" = 1.27
  dimension "d66" = 2.54
  constraints: 24 end point, 8 point on circle, 4 centre point, 4 midpoint, 4 parallel, 2 horizontal, 2 perpendicular, 2 point on line, 7 other
  measures "d62" distance between parallel lines of L2 L4
  measures "d63" distance of L10.end L9.end
  measures "d64" distance of L9.end L8.end
  measures "d65" distance of L13.end L14.end
  measures "d66" distance of L12.end L13.end
extrude "Extrusion15" add sketch "Sketch10" along normal blind 3.556 contours L10 L9 L8 L4 | L6 L12 L13 L14
sketch "Sketch11" plane through (-6.3591, 9.6171, 6.8256) normal (0, 0, -1) x (-1, 0, 0)
  line L0 (-9.0643, 1.73) -> (-7.7943, 1.73) projected
  line L1 (-7.7943, 1.73) -> (-7.7943, 4.27) projected
  line L2 (-7.7943, 4.27) -> (-9.0643, 4.27) projected
  line L3 (-9.0643, 4.27) -> (-9.0643, 1.73) projected
  line L4 (-0.2703, 4.27) -> (-1.5403, 4.27) projected
  line L5 (-1.5403, 4.27) -> (-1.5403, 1.73) projected
  line L6 (-1.5403, 1.73) -> (-0.2703, 1.73) projected
  line L7 (-0.2703, 1.73) -> (-0.2703, 4.27) projected
  line L8 (-7.7943, 4.27) -> (-7.4133, 4.27)
  line L9 (-7.4133, 4.27) -> (-7.4133, 1.73)
  line L10 (-7.4133, 1.73) -> (-7.7943, 1.73)
  line L11 (-7.7943, 1.73) -> (-7.7943, 4.27)
  line L12 (-1.5403, 4.27) -> (-1.9213, 4.27)
  line L13 (-1.9213, 4.27) -> (-1.9213, 1.73)
  line L14 (-1.9213, 1.73) -> (-1.5403, 1.73)
  line L15 (-1.5403, 1.73) -> (-1.5403, 4.27)
  point P0 (-6.3591, -9.6171)
  point P1 (-1.7308, 1.73)
  point P2 (-7.7943, 1.73)
  dimension "d69" = 0.381
  dimension "d70" = 0.381
  constraints: 16 end point, 4 parallel, 2 horizontal, 2 perpendicular, 1 horizontal alignment, 1 midpoint, 1 point on line
  measures "d69" distance of L9.end L10.end
  measures "d70" distance of L14.end L13.end
extrude "Extrusion16" add sketch "Sketch11" along normal blind 0.762
chamfer "Chamfer4" distance 0.508 angle 45 2 edges at (1.0541, 12.6171, 6.0636) (-4.4379, 12.6171, 6.0636)
body "Solid1"
